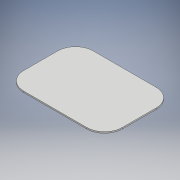
# Autodesk Inventor part: Game_ColonyPort
Saved by Autodesk Inventor 2018 (Build 220112000, 112)
## iProperties
Created: 2021-04-21
Part Number: Game_ColonyPort
Material: Generic
Document SubType Name: Modeling
Designer: Bradley
Density: 1 g/cm^3
Appearance: Default
Author: Bradley
Autodesk Inventor part; units mm, degrees
ref_plane "YZ Plane" through (0, 0, 0) normal (1, 0, 0) x (0, 1, 0)
ref_plane "XZ Plane" through (0, 0, 0) normal (0, 1, 0) x (-1, 0, 0)
ref_plane "XY Plane" through (0, 0, 0) normal (0, 0, 1) x (1, 0, 0)
sketch "Sketch1" plane through (0, 0, 0) normal (0, 0, 1) x (1, 0, 0)
  line L0 (-44.5, -49) -> (44.5, -49)
  line L1 (69.5, -24) -> (69.5, 24)
  line L2 (44.5, 49) -> (-44.5, 49)
  line L3 (-69.5, 24) -> (-69.5, -24)
  line L4 (-69.5, -49) -> (69.5, 49) construction
  line L5 (69.5, -49) -> (-69.5, 49) construction
  arc A0 (69.5, 24) -> (44.5, 49) centre (44.5, 24) ccw
  arc A1 (44.5, -49) -> (69.5, -24) centre (44.5, -24) ccw
  arc A2 (-69.5, -24) -> (-44.5, -49) centre (-44.5, -24) ccw
  arc A3 (-44.5, 49) -> (-69.5, 24) centre (-44.5, 24) ccw
  point P0 (0, 0)
  dimension "d0" = 139
  dimension "d1" = 98
  dimension "d2" = 25
  constraints: 12 end point, 8 point on circle, 8 point on line, 8 tangent, 4 centre point, 3 equal radius, 2 midpoint, 2 parallel, 1 horizontal, 1 perpendicular
  measures "d0" distance of L5.end L4.end
  measures "d1" distance of L4.end L5.start
  measures "d2" radius of A0
extrude "Extrusion1" add sketch "Sketch1" along normal mid plane 2
body "Solid1"
